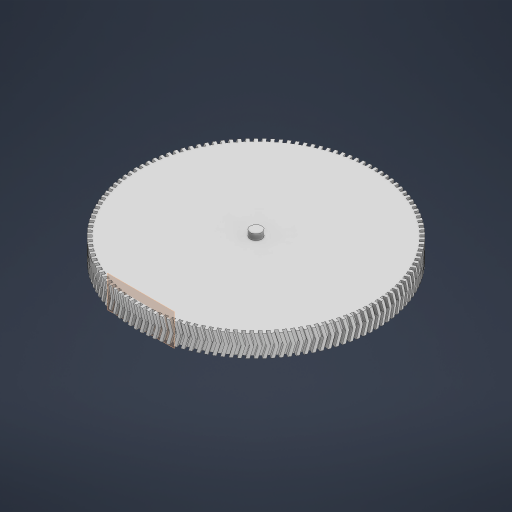
# Autodesk Inventor part: y-axis-gear
Saved by Autodesk Inventor 2023 (Build 270158000, 158)
## iProperties
Created: 2022-05-14
Part Number: y-axis-gear
Material: Generic
Document SubType Name: Modeling
Designer: jayso
Density: 1 g/cm^3
Appearance: Default
Author: jayso
Autodesk Inventor part; units mm, degrees
ref_plane "YZ Plane" through (0, 0, 0) normal (1, 0, 0) x (0, 1, 0)
ref_plane "XZ Plane" through (0, 0, 0) normal (0, 1, 0) x (-1, 0, 0)
sketch "Sketch3" plane through (0, 0, 0) normal (0, 1, 0) x (-1, 0, 0)
  circle A0 centre (0, 0) radius 80
  dimension "d0" = 160
  constraints: 1 centre point, 1 coincident
  measures "d0" diameter of A0
extrude "Extrusion1" add sketch "Sketch3" along normal blind 15
ref_plane "Work Plane1" through (0, 0, 79.5) normal (0, 0, 1) x (1, 0, 0)
sketch "Sketch8" plane through (0, 0, 79.5) normal (0, 0, 1) x (1, 0, 0)
  line L0 (80, 15) -> (-80, 15) projected
  line L1 (0, 15) -> (0, 0)
  line L2 (0, 0) -> (2, 0)
  line L3 (80, 0) -> (-80, 0) projected
  line L4 (0, 7.5) -> (2, 7.5)
  line L5 (2, 7.5) -> (0, 0)
  line L6 (2, 7.5) -> (0, 15)
  line L7 (0, 15) -> (-2, 15)
  line L8 (-2, 15) -> (0, 7.5)
  line L9 (0, 7.5) -> (-2, 0)
  dimension "d4" = 2
  dimension "d5" = 2
  dimension "d6" = 2
  constraints: 16 end point, 3 point on line, 2 midpoint, 1 horizontal, 1 parallel, 1 vertical
  measures "d4" distance of L1.end L2.end
  measures "d5" distance of L4.start L4.end
  measures "d6" distance of L1.start L7.end
extrude "Extrusion2" add sketch "Sketch8" along normal blind 3
pattern_circular "Circular Pattern1" count 126 over 360 about axis through (0, 0, 0) along (0, 1, 0) of "Extrusion2"
sketch "Sketch10" plane through (0, 15, 0) normal (0, 1, 0) x (1, 0, 0)
  circle A0 centre (0, 0) radius 2.5
  line L0 (0, 2.5) -> (0, -1.9)
  line L1 (0, -1.9) -> (1.6248, -1.9)
  line L2 (-1.6248, -1.9) -> (0, -1.9)
  dimension "d17" = 5
  dimension "d18" = 4.4
  constraints: 6 end point, 3 point on circle, 1 centre point, 1 coincident, 1 horizontal, 1 perpendicular, 1 vertical
  measures "d17" diameter of A0
  measures "d18" distance of L0.start L0.end
extrude "Extrusion3" cut sketch "Sketch10" against normal blind 21 contours A0 L1 L0 | L0 L2 A0
sketch "Sketch13" plane through (0, 0, 0) normal (0, -1, 0) x (1, 0, 0)
  circle A0 centre (0, 0) radius 4
  dimension "d21" = 8
  constraints: 1 centre point, 1 coincident
  measures "d21" diameter of A0
extrude "Extrusion4" add sketch "Sketch13" along normal blind 15 and the other way blind 15
sketch "Sketch14" plane through (0, 15, 0) normal (0, 1, 0) x (1, 0, 0)
  arc A0 (1.6248, -1.9) -> (-1.6248, -1.9) centre (0, 0) ccw projected
  circle A1 centre (0, 0) radius 4
  dimension "d24" = 8
  constraints: 1 centre point, 1 coincident
  measures "d24" diameter of A1
extrude "Extrusion5" add sketch "Sketch14" along normal blind 4
body "Solid1"
